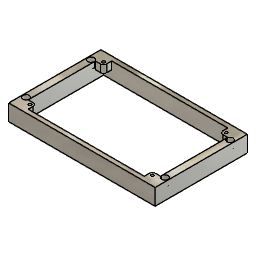
EncaixeEcraPoncha (Autodesk Fusion 360 design; units mm, degrees)
Autodesk Fusion 360 part; units mm, degrees
note: some values were not read from the file. Set by a fixed rule: which sketch regions a step uses.
sketch "Sketch1" plane through (0, 0, 0) normal (0, 1, 0) x (1, 0, 0)
  line L0 (56.5, -34) -> (-56.5, -34)
  line L1 (-56.5, -34) -> (-56.5, 34)
  line L2 (-56.5, 34) -> (56.5, 34)
  line L3 (56.5, 34) -> (56.5, -34)
  line L4 (56.5, -34) -> (-56.5, 34) construction
  line L5 (-56.5, -34) -> (56.5, 34) construction
  line L6 (64, 30) -> (-64, 30)
  line L7 (-64, 30) -> (-64, -30)
  line L8 (-64, -30) -> (64, -30)
  line L9 (64, -30) -> (64, 30)
  line L10 (64, 30) -> (-64, -30) construction
  line L11 (-64, 30) -> (64, -30) construction
  circle A0 centre (64, 30) radius 1.25
  line L12 (60.5, -38) -> (-60.5, -38)
  line L13 (-60.5, -38) -> (-60.5, 38)
  line L14 (-60.5, 38) -> (60.5, 38)
  line L15 (60.5, 38) -> (60.5, -38)
  line L16 (60.5, -38) -> (-60.5, 38) construction
  line L17 (-60.5, -38) -> (60.5, 38) construction
  circle A1 centre (-56.5, 34) radius 1.25
  circle A2 centre (-56.5, 34) radius 3
  circle A3 centre (56.5, 34) radius 1.25
  circle A4 centre (56.5, 34) radius 3
  circle A5 centre (56.5, -34) radius 1.25
  circle A6 centre (56.5, -34) radius 3
  circle A7 centre (-56.5, -34) radius 1.25
  circle A8 centre (-56.5, -34) radius 3
  circle A9 centre (64, -30) radius 1.25
  circle A10 centre (-64, -30) radius 1.25
  circle A11 centre (-64, 30) radius 1.25
  circle A12 centre (-64, 30) radius 3
  circle A13 centre (64, 30) radius 3
  circle A14 centre (64, -30) radius 3
  circle A15 centre (-64, -30) radius 3
  line L18 (61, -38.5) -> (-61, -38.5)
  line L19 (-61, -38.5) -> (-61, 38.5)
  line L20 (-61, 38.5) -> (61, 38.5)
  line L21 (61, 38.5) -> (61, -38.5)
  line L22 (61, -38.5) -> (-61, 38.5) construction
  line L23 (-61, -38.5) -> (61, 38.5) construction
  line L24 (67.5, -42.5) -> (-67.5, -42.5)
  line L25 (-67.5, -42.5) -> (-67.5, 42.5)
  line L26 (-67.5, 42.5) -> (67.5, 42.5)
  line L27 (67.5, 42.5) -> (67.5, -42.5)
  line L28 (67.5, -42.5) -> (-67.5, 42.5) construction
  line L29 (-67.5, -42.5) -> (67.5, 42.5) construction
  dimension "d1" = 113
  dimension "d2" = 68
  dimension "d3" = 128
  dimension "d4" = 60
  dimension "d5" = 2.5
  dimension "d6" = 121
  dimension "d7" = 76
  dimension "d8" = 2.5
  dimension "d9" = 6
  dimension "d10" = 2.5
  dimension "d11" = 6
  dimension "d12" = 2.5
  dimension "d13" = 6
  dimension "d14" = 2.5
  dimension "d15" = 6
  dimension "d16" = 2.5
  dimension "d17" = 2.5
  dimension "d18" = 2.5
  dimension "d19" = 6
  dimension "d20" = 6
  dimension "d21" = 6
  dimension "d22" = 6
  dimension "d25" = 122
  dimension "d26" = 77
  dimension "d27" = 135
  dimension "d28" = 85
  constraint horizontal L0
  constraint perpendicular L0 L1
  constraint parallel L0 L2
  constraint parallel L1 L3
  constraint coincident L4 origin
  constraint coincident L5 origin
  constraint horizontal L6
  constraint perpendicular L6 L7
  constraint parallel L6 L8
  constraint parallel L7 L9
  constraint coincident L10 origin
  constraint coincident L11 origin
  constraint coincident L6.start L9.end
  constraint horizontal L12
  constraint perpendicular L12 L13
  constraint parallel L12 L14
  constraint parallel L13 L15
  constraint coincident L16 origin
  constraint coincident L17 origin
  constraint coincident L1.end L2.start
  constraint concentric A1 A2
  constraint coincident L2.end L3.start
  constraint concentric A3 A4
  constraint coincident L0.start L3.end
  constraint concentric A5 A6
  constraint coincident L0.end L1.start
  constraint concentric A7 A8
  constraint coincident L8.end L9.start
  constraint coincident L7.end L8.start
  constraint coincident L6.end L7.start
  constraint concentric A11 A12
  constraint concentric A0 A13
  constraint concentric A9 A14
  constraint concentric A10 A15
  constraint horizontal L18
  constraint perpendicular L18 L19
  constraint parallel L18 L20
  constraint parallel L19 L21
  constraint coincident L22 origin
  constraint coincident L23 origin
  constraint horizontal L24
  constraint perpendicular L24 L25
  constraint parallel L24 L26
  constraint parallel L25 L27
  constraint coincident L28 origin
  constraint coincident L29 origin
  measures "d1" distance of L1.end L2.end
  measures "d2" distance of L0.end L1.end
  measures "d3" distance of L7.end L8.end
  measures "d4" distance of L6.end L7.end
  measures "d5" diameter of A0
  measures "d6" distance of L13.end L14.end
  measures "d7" distance of L12.end L13.end
  measures "d8" diameter of A1
  measures "d9" diameter of A2
  measures "d10" diameter of A3
  measures "d11" diameter of A4
  measures "d12" diameter of A5
  measures "d13" diameter of A6
  measures "d14" diameter of A7
  measures "d15" diameter of A8
  measures "d16" diameter of A9
  measures "d17" diameter of A10
  measures "d18" diameter of A11
  measures "d19" diameter of A12
  measures "d20" diameter of A13
  measures "d21" diameter of A14
  measures "d22" diameter of A15
  measures "d25" distance of L19.end L20.end
  measures "d26" distance of L18.end L19.end
extrude "Extrude1" add sketch "Sketch1" along normal blind 8 contours L0 L1 A7 A8 | L0 L1 A7 A8 | L0 L3 A5 A6 | L0 L3 A5 A6 | L1 L2 A1 A2 | L1 L2 A1 A2 | L2 L3 A3 A4 | L2 L3 A3 A4 makes body 1 at (-53.5149, 5.3333, -34.2987) makes body 2 at (-53.5149, 5.3333, 33.7013) makes body 3 at (59.4851, 5.3333, -34.2987) makes body 4 at (59.4851, 5.3333, 33.7013)
extrude "Extrude2" add sketch "Sketch1" along normal blind 15 separate body contours L7 A12 A15 L19 | L9 A13 A14 L21 | L24 L25 L26 L27 makes body 5
extrude "Extrude3" add sketch "Sketch1" along normal blind 10 separate body contours L7 L8 A10 A15 | L7 L8 A10 A15 | L8 L9 A9 A14 | L8 L9 A9 A14 | L6 L7 A11 A12 | L6 L7 A11 A12 | L6 L9 A0 A13 | L6 L9 A0 A13 makes body 6 at (64.5209, 6.6667, 32.9544) makes body 7 at (-61.0149, 6.6667, 29.7013) makes body 8 at (64.9555, 3.3333, -32.8438) makes body 9 at (-61.0149, 6.6667, -30.2987)
sketch "Sketch2" plane through (0, 15, 0) normal (0, 1, 0) x (-1, 0, 0)
  line L0 (61, -38.5) -> (-61, -38.5)
  line L1 (-61, -38.5) -> (-61, -30)
  circle A0 centre (-64, -30) radius 3
  line L2 (-61, -30) -> (-61, 30)
  circle A1 centre (-64, 30) radius 3
  line L3 (-61, 30) -> (-61, 38.5)
  line L4 (-61, 38.5) -> (61, 38.5)
  line L5 (61, 38.5) -> (61, 30)
  circle A2 centre (64, 30) radius 3
  line L6 (61, 30) -> (61, -30)
  circle A3 centre (64, -30) radius 3
  line L7 (61, -30) -> (61, -38.5)
  line L8 (-67.5, -42.5) -> (67.5, -42.5)
  line L9 (67.5, -42.5) -> (67.5, 42.5)
  line L10 (67.5, 42.5) -> (-67.5, 42.5)
  line L11 (-67.5, 42.5) -> (-67.5, -42.5)
  line L12 (-56.5, -34) -> (56.5, -34)
  line L13 (56.5, -34) -> (56.5, 34)
  line L14 (56.5, 34) -> (-56.5, 34)
  line L15 (-56.5, 34) -> (-56.5, -34)
  line L16 (-56.5, -34) -> (56.5, 34) construction
  line L17 (56.5, -34) -> (-56.5, 34) construction
  circle A4 centre (56.5, -34) radius 1.25
  circle A5 centre (56.5, -34) radius 3
  line L18 (56.5, -31) -> (61, -31)
  line L19 (53.5, -34) -> (53.5, -38.5)
  line L20 (0, 0) -> (0, -46.2304) construction
  line L21 (0, 0) -> (-40.9385, 0) construction
  line L22 (-53.5, -34) -> (-53.5, -38.5)
  circle A6 centre (-56.5, -34) radius 3
  circle A7 centre (-56.5, -34) radius 1.25
  line L23 (-56.5, -31) -> (-61, -31)
  line L24 (56.5, 31) -> (61, 31)
  circle A8 centre (56.5, 34) radius 3
  circle A9 centre (56.5, 34) radius 1.25
  line L25 (53.5, 34) -> (53.5, 38.5)
  line L26 (-56.5, 31) -> (-61, 31)
  circle A10 centre (-56.5, 34) radius 3
  circle A11 centre (-56.5, 34) radius 1.25
  line L27 (-53.5, 34) -> (-53.5, 38.5)
  dimension "d33" = 113
  dimension "d34" = 68
  dimension "d35" = 2.5
  dimension "d36" = 6
  constraint horizontal L12
  constraint perpendicular L12 L13
  constraint parallel L12 L14
  constraint parallel L13 L15
  constraint coincident L16 L20.start
  constraint coincident L17 L20.start
  constraint coincident L20.start L21.start
  constraint coincident L12.end L13.start
  constraint concentric A4 A5
  constraint coincident A5 L18.start
  constraint coincident L13 L18.start
  constraint coincident L7 L18.end
  constraint tangent A5 L18
  constraint coincident A5 L19.start
  constraint coincident L12 L19.start
  constraint coincident L0 L19.end
  constraint tangent A5 L19
  constraint perpendicular L8 L20
  constraint perpendicular L20 L21
  constraint symmetric A4 L20 A7
  constraint symmetric A5 L20 A6
  constraint symmetric L18.start L20 L23.start
  constraint symmetric L18.end L20 L23.end
  constraint symmetric L19.start L20 L22.start
  constraint symmetric L19.end L20 L22.end
  constraint symmetric A4 L21 A9
  constraint symmetric A5 L21 A8
  constraint symmetric L18.start L21 L24.start
  constraint symmetric L18.end L21 L24.end
  constraint symmetric L19.start L21 L25.start
  constraint symmetric L19.end L21 L25.end
  constraint symmetric L21 L22.start L27.start
  constraint symmetric L21 L22.end L27.end
  constraint symmetric L21 A6 A10
  constraint symmetric L21 A7 A11
  constraint symmetric L21 L23.start L26.start
  constraint symmetric L21 L23.end L26.end
  measures "d33" distance of L13.end L14.end
  measures "d34" distance of L12.end L13.end
  measures "d35" diameter of A4
  measures "d36" diameter of A5
extrude "Extrude4" add sketch "Sketch2" against normal blind 7 separate body contours L0 L7 A5 L18 L19 | L0 L1 L22 A6 L23 | L12 L13 A4 A5 | L12 L13 A4 A5 | L12 L15 A6 A7 | L12 L15 A6 A7 | L13 L14 A8 A9 | L4 L5 L24 A8 L25 | L13 L14 A8 A9 | L14 L15 A10 A11 | L3 L4 L26 A10 L27 | L14 L15 A10 A11 makes body 10 at (-57.4576, 10.3333, 34.8035) makes body 11 at (55.5036, 10.3333, -34.7548) makes body 12 at (57.6746, 12.6667, 33.5725) makes body 13 at (-55.3254, 10.3333, -33.5725)
combine "Combine1" operation add target body 13 tool bodies 12 11 10 5 9 8 7 6
hidden bodies 1 2 3 4
